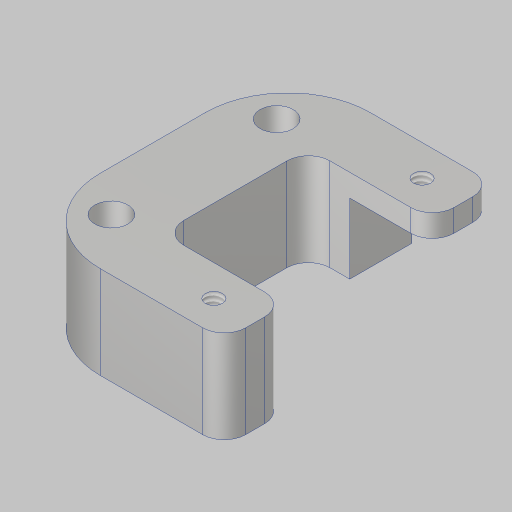
# Autodesk Inventor part: GP7-006
Saved by Autodesk Inventor 2023.5 (Build 275446000, 446)
## iProperties
Created: 2025-02-25
Part Number: GP7-006
Material: Aluminum 6061
Document SubType Name: Modeling
Designer: slick
Density: 2.7 g/cm^3
Appearance: Aluminum - Flat
Author: slick
Autodesk Inventor part; units mm, degrees
ref_plane "YZ Plane" through (0, 0, 0) normal (1, 0, 0) x (0, 1, 0)
ref_plane "XZ Plane" through (0, 0, 0) normal (0, 1, 0) x (-1, 0, 0)
ref_plane "XY Plane" through (0, 0, 0) normal (0, 0, 1) x (1, 0, 0)
sketch "Sketch1" plane through (0, 0, 0) normal (1, 0, 0) x (0, 1, 0)
  line L0 (0, 20.7625) -> (0, -20.7625)
  line L1 (0, 20.7625) -> (14.224, 20.7625)
  line L2 (14.224, 20.7625) -> (14.224, 11.2375)
  line L3 (14.224, 11.2375) -> (6.35, 11.2375)
  line L4 (6.35, 11.2375) -> (6.35, -11.2375)
  line L5 (6.35, -11.2375) -> (14.224, -11.2375)
  line L6 (14.224, -11.2375) -> (14.224, -20.7625)
  line L7 (14.224, -20.7625) -> (0, -20.7625)
  point P0 (0, 0)
  point P1 (0, 0)
  point P2 (14.224, -16)
  point P3 (14.224, 16)
  dimension "d1" = 32
  dimension "d2" = 7.874
  dimension "d4" = 6.35
  dimension "d5" = 9.525
  constraints: 16 end point, 6 perpendicular, 3 midpoint, 2 coincident, 1 collinear, 1 horizontal, 1 vertical, 1 vertical alignment
  measures "d1" distance of point (14.224, -16) point (14.224, 16)
  measures "d2" distance of L2.end L3.end
  measures "d4" distance between parallel lines of L0 L4
  measures "d5" distance between parallel lines of L3 L1
extrude "Extrusion1" add sketch "Sketch1" along normal blind 31.75
sketch "Sketch2" plane through (0, 14.224, 20.7625) normal (0, 1, 0) x (1, 0, 0)
  line L0 (0, 9.525) -> (31.75, 9.525) construction
  line L1 (31.75, 9.525) -> (31.75, 0) construction
  line L2 (31.75, 0) -> (0, 0) construction
  line L3 (0, 0) -> (0, 9.525) construction
  line L4 (0, 41.525) -> (31.75, 41.525) construction
  line L5 (31.75, 41.525) -> (31.75, 32) construction
  line L6 (31.75, 32) -> (0, 32) construction
  line L7 (0, 32) -> (0, 41.525) construction
  point P0 (0, 20.7625)
  point P1 (25.4, 4.7625)
  point P2 (25.4, 36.7625)
  point P3 (31.75, 4.7625)
  point P4 (31.75, 36.7625)
  dimension "d8" = 6.35
  constraints: 2 horizontal alignment, 2 midpoint, 1 vertical alignment
  measures "d8" distance from line of L1 point (25.4, 4.762)
hole "Hole1" at (25.4, 14.224, 16) at (25.4, 14.224, -16) direction (0, -1, 0) diameter 2.6416 end through all thread size "6-32 UNC" class "2B" standard "ANSI Unified Screw Threads"
sketch "Sketch4" plane through (0, 6.35, 11.2375) normal (0, 1, 0) x (1, 0, 0)
  circle A0 centre (25.4, -4.7625) radius 1.3208 construction
  circle A1 centre (25.4, 27.2375) radius 1.3208 construction
  line L0 (0, 32) -> (31.75, 32) construction
  line L1 (31.75, 32) -> (31.75, 22.475) construction
  line L2 (31.75, 22.475) -> (0, 22.475) construction
  line L3 (0, 0) -> (0, 22.475) construction
  line L4 (0, 0) -> (31.75, 0) construction
  line L5 (31.75, 0) -> (31.75, -9.525) construction
  line L6 (31.75, -9.525) -> (0, -9.525) construction
  line L7 (0, -9.525) -> (0, 0) construction
  line L8 (0, 22.475) -> (0, 32) construction
  line L9 (31.75, 22.475) -> (31.75, 0) construction
  line L10 (0, 22.475) -> (31.75, 22.475) construction
  line L11 (31.75, 0) -> (12.7, 0)
  line L12 (12.7, 0) -> (12.7, 22.475)
  line L13 (12.7, 22.475) -> (31.75, 22.475)
  line L14 (31.75, 22.475) -> (31.75, 0)
  point P0 (0, 11.2375)
  point P1 (14.7922, 22.475)
  dimension "d25" = 19.05
  constraints: 8 end point, 2 parallel, 1 horizontal, 1 perpendicular, 1 point on line
  measures "d25" distance between parallel lines of L9 L12
extrude "Extrusion2" cut sketch "Sketch4" along normal mid plane 38.1
sketch "Sketch5" plane through (0, 14.224, 20.7625) normal (0, 1, 0) x (1, 0, 0)
  line L0 (0, 0) -> (0, 41.525) construction
  line L1 (0, 41.525) -> (31.75, 41.525) construction
  line L2 (0, 41.525) -> (12.7, 41.525)
  line L3 (12.7, 41.525) -> (12.7, 0.1925)
  line L4 (12.7, 0.1925) -> (0, 0.1925)
  line L5 (0, 0.1925) -> (0, 41.525)
  line L6 (12.7, 9.525) -> (12.7, 32) construction
  point P0 (0, 20.7625)
  constraints: 8 end point, 2 parallel, 1 collinear, 1 horizontal, 1 perpendicular
extrude "Extrusion3" add sketch "Sketch5" against normal up to surface (7.874 mm away)
sketch "Sketch6" plane through (0, 14.224, 20.7625) normal (0, 1, 0) x (1, 0, 0)
  line L0 (6.35, 8.0625) -> (6.35, 33.4625) construction
  line L1 (0, 41.525) -> (0, 0) construction
  point P0 (0, 20.7625)
  point P1 (6.35, 20.7625)
  point P2 (0, 20.7625)
  dimension "d30" = 6.35
  dimension "d31" = 25.4
  constraints: 2 end point, 2 midpoint, 1 horizontal alignment, 1 vertical, 1 vertical alignment
  measures "d30" distance between parallel lines of L1 L0
  measures "d31" distance of L0.start L0.end
hole "Hole3" at (6.35, 14.224, 12.7) at (6.35, 14.224, -12.7) direction (0, -1, 0) diameter 5.1054 end through all clearance for "Flat Head Machine Screw (82)" size "#10" standard "Ansi Unified Screw Threads"
fillet "Fillet1" radius 12.7 2 edges at (0, 7.112, -20.7625) (0, 7.112, 20.7625)
fillet "Fillet2" radius 3.302 6 edges at (12.7, 7.112, -11.2375) (12.7, 7.112, 11.2375) (31.75, 7.112, 20.7625) (31.75, 7.112, 11.2375) (31.75, 7.112, -11.2375) (31.75, 7.112, -20.7625)
sketch "Sketch7" plane through (0, 0, -8.0625) normal (0, -1, 0) x (1, 0, 0)
  arc A0 (16.002, 19.3) -> (12.7, 15.998) centre (16.002, 15.998) ccw construction
  line L0 (12.7, 15.998) -> (12.7, 0.127) construction
  arc A1 (12.7, 0.127) -> (16.002, -3.175) centre (16.002, 0.127) ccw construction
  line L1 (16.002, -3.175) -> (28.448, -3.175) construction
  arc A2 (31.75, -6.477) -> (28.448, -3.175) centre (28.448, -6.477) ccw projected
  line L2 (31.75, -6.477) -> (31.75, -9.398) projected
  arc A3 (28.448, -12.7) -> (31.75, -9.398) centre (28.448, -9.398) ccw projected
  line L3 (28.448, -12.7) -> (12.7, -12.7) construction
  arc A4 (0, 0) -> (12.7, -12.7) centre (12.7, 0) ccw construction
  line L4 (0, 0) -> (0, 16.125) construction
  arc A5 (12.7, 28.825) -> (0, 16.125) centre (12.7, 16.125) ccw construction
  line L5 (12.7, 28.825) -> (28.448, 28.825) construction
  arc A6 (31.75, 25.523) -> (28.448, 28.825) centre (28.448, 25.523) ccw construction
  line L6 (31.75, 25.523) -> (31.75, 22.602) construction
  arc A7 (28.448, 19.3) -> (31.75, 22.602) centre (28.448, 22.602) ccw construction
  line L7 (28.448, 19.3) -> (16.002, 19.3) construction
  circle A8 centre (6.35, 20.7625) radius 2.5527 construction
  circle A9 centre (6.35, -4.6375) radius 2.5527 construction
  circle A10 centre (25.4, 24.0625) radius 1.3208 construction
  circle A11 centre (25.4, -7.9375) radius 1.3208 projected
  line L8 (12.7, -12.7) -> (28.448, -12.7) construction
  line L9 (28.448, -12.7) -> (19.05, -12.7)
  line L10 (19.05, -12.7) -> (19.05, -3.175)
  line L11 (16.002, -3.175) -> (28.448, -3.175) construction
  line L12 (19.05, -3.175) -> (28.448, -3.175)
  point P0 (0, 8.0625)
  dimension "d41" = 12.7
  constraints: 6 end point, 2 point on line, 1 perpendicular
  measures "d41" distance between parallel lines of L2 L10
extrude "Extrusion4" cut sketch "Sketch7" against normal blind 10.795
body "Solid1"
